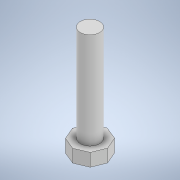
# Autodesk Inventor part: Screw 3mm
Saved by Autodesk Inventor 2022 (Build 260153000, 153)
## iProperties
Created: 2022-06-15
Part Number: Screw 3mm
Material: Generic
Document SubType Name: Modeling
Designer: chait
Density: 1 g/cm^3
Appearance: Default
Author: chait
Autodesk Inventor part; units mm, degrees
ref_plane "YZ Plane" through (0, 0, 0) normal (1, 0, 0) x (0, 1, 0)
ref_plane "XZ Plane" through (0, 0, 0) normal (0, 1, 0) x (-1, 0, 0)
ref_plane "XY Plane" through (0, 0, 0) normal (0, 0, 1) x (1, 0, 0)
sketch "Sketch1" plane through (0, 0, 0) normal (0, 1, 0) x (-1, 0, 0)
  line L0 (-1.8907, -1.9359) -> (-2.7058, -0.032)
  line L1 (-2.7058, -0.032) -> (-1.9359, 1.8907)
  line L2 (-1.9359, 1.8907) -> (-0.032, 2.7058)
  line L3 (-0.032, 2.7058) -> (1.8907, 1.9359)
  line L4 (1.8907, 1.9359) -> (2.7058, 0.032)
  line L5 (2.7058, 0.032) -> (1.9359, -1.8907)
  line L6 (1.9359, -1.8907) -> (0.032, -2.7058)
  line L7 (0.032, -2.7058) -> (-1.8907, -1.9359)
  point P0 (0, 0)
  point P1 (0, 0)
  dimension "d0" = 5
  constraints: 16 end point, 1 coincident, 17 other
  measures "d0" distance from line of L6.end L3
extrude "Extrusion1" add sketch "Sketch1" along normal blind 2
sketch "Sketch2" plane through (0, 2, 0) normal (0, 1, 0) x (1, 0, 0)
  circle A0 centre (0, 0) radius 1.5
  dimension "d3" = 3
  constraints: 1 centre point, 1 coincident
  measures "d3" diameter of A0
extrude "Extrusion2" add sketch "Sketch2" along normal blind 15
body "Solid1"
